Autodesk Inventor part; units mm, degrees
(part 4 of 4)
  line L152 (26.499495, -98.072286) -> (23.480041, -98.072286)
  line L153 (49.613875, -90.119995) -> (49.613875, -91.883884)
  line L154 (3.752764, -90.119995) -> (49.613875, -90.119995)
  line L155 (3.752764, -91.883884) -> (3.752764, -90.119995)
  line L156 (49.613875, -91.883884) -> (3.752764, -91.883884)
  line L157 (48.511932, -114.397733) -> (43.700857, -114.397733)
  spline S115 degree 3 poles (48.511932, -112.845889) (48.92121, -112.845889) (49.203363, -113.170245) (49.203363, -113.621725) (49.203363, -114.073205) (48.92121, -114.397733) (48.511932, -114.397733) knots 0 0 0 0 0.5 0.5 0.5 1 1 1 1
  line L158 (43.785606, -112.845889) -> (48.511932, -112.845889)
  spline S116 degree 3 poles (41.14718, -110.390914) (41.14718, -111.900555) (42.177091, -112.845889) (43.785606, -112.845889) knots 0 0 0 0 1 1 1 1
  spline S117 degree 3 poles (43.785606, -107.935939) (42.191216, -107.935939) (41.14718, -108.867148) (41.14718, -110.390914) knots 0 0 0 0 1 1 1 1
  line L159 (48.511932, -107.935939) -> (43.785606, -107.935939)
  spline S118 degree 3 poles (48.511932, -106.383924) (48.92121, -106.383924) (49.203363, -106.708452) (49.203363, -107.159931) (49.203363, -107.611411) (48.92121, -107.935939) (48.511932, -107.935939) knots 0 0 0 0 0.5 0.5 0.5 1 1 1 1
  line L160 (43.700857, -106.383924) -> (48.511932, -106.383924)
  spline S119 degree 3 poles (43.700857, -114.397733) (41.358881, -114.397733) (39.637539, -112.902217) (39.637539, -110.390914) (39.637539, -107.865487) (41.358881, -106.383924) (43.700857, -106.383924) knots 0 0 0 0 0.5 0.5 0.5 1 1 1 1
  spline S120 degree 3 poles (48.102827, -98.77767) (48.89296, -99.088073) (49.189238, -99.511303) (49.189238, -100.146234) knots 0 0 0 0 1 1 1 1
  line L161 (40.977853, -95.814887) -> (48.102827, -98.77767)
  spline S121 degree 3 poles (40.427671, -95.687763) (40.611123, -95.673811) (40.780449, -95.730138) (40.977853, -95.814887) knots 0 0 0 0 1 1 1 1
  spline S122 degree 3 poles (40.30072, -97.239779) (39.919692, -97.084577) (39.722288, -96.844799) (39.722288, -96.477896) (39.722288, -96.026416) (40.018566, -95.716013) (40.427671, -95.687763) knots 0 0 0 0 0.5 0.5 0.5 1 1 1 1
  line L162 (42.092514, -97.973412) -> (40.30072, -97.239779)
  line L163 (42.092514, -102.389508) -> (42.092514, -97.973412)
  line L164 (40.314844, -103.109016) -> (42.092514, -102.389508)
  spline S123 degree 3 poles (40.921526, -104.590407) (40.738074, -104.661031) (40.582873, -104.703406) (40.470046, -104.703406) (40.032691, -104.703406) (39.722288, -104.350628) (39.722288, -103.885024) (39.722288, -103.546371) (39.933817, -103.264217) (40.314844, -103.109016) knots 0 0 0 0 0.33333333 0.33333333 0.33333333 0.66666667 0.66666667 0.66666667 1 1 1 1
  line L165 (48.102827, -101.627625) -> (40.921526, -104.590407)
  spline S124 degree 3 poles (49.189238, -100.244936) (49.189238, -100.893992) (48.89296, -101.303097) (48.102827, -101.627625) knots 0 0 0 0 1 1 1 1
  line L166 (49.189238, -100.146234) -> (49.189238, -100.244936)
  line L167 (30.611044, -74.123016) -> (44.760051, -74.123016)
  line L168 (30.611044, -77.145915) -> (30.611044, -74.123016)
  line L169 (44.760051, -77.145915) -> (30.611044, -77.145915)
  line L170 (44.760051, -82.150088) -> (44.760051, -77.145915)
  line L171 (47.757456, -82.150088) -> (44.760051, -82.150088)
  line L172 (47.757456, -69.134173) -> (47.757456, -82.150088)
  line L173 (47.757456, -60.446504) -> (47.757456, -69.134173)
  spline S125 degree 3 poles (37.876061, -60.751395) (37.876061, -56.179064) (40.441624, -55.112118) (42.82942, -55.112118) (45.674552, -55.112118) (47.757456, -56.636228) (47.757456, -60.446504) knots 0 0 0 0 0.5 0.5 0.5 1 1 1 1
  line L174 (37.876061, -64.739609) -> (37.876061, -60.751395)
  spline S126 degree 3 poles (33.608449, -65.069822) (33.608449, -66.695562) (34.497628, -67.432124) (35.742341, -67.432124) (36.85993, -67.432124) (37.876061, -66.847836) (37.876061, -64.739609) knots 0 0 0 0 0.5 0.5 0.5 1 1 1 1
  line L175 (33.608449, -55.417009) -> (33.608449, -65.069822)
  line L176 (30.611044, -55.417009) -> (33.608449, -55.417009)
  line L177 (30.611044, -64.968192) -> (30.611044, -55.417009)
  spline S127 degree 3 poles (40.6957, -64.663301) (40.6957, -69.337262) (38.104643, -70.429701) (35.640711, -70.429701) (32.744764, -70.429701) (30.611044, -68.880097) (30.611044, -64.968192) knots 0 0 0 0 0.5 0.5 0.5 1 1 1 1
  line L178 (40.6957, -60.649764) -> (40.6957, -64.663301)
  spline S128 degree 3 poles (44.760051, -60.344873) (44.760051, -58.795442) (43.921859, -58.109523) (42.727962, -58.109523) (41.686337, -58.109523) (40.6957, -58.642996) (40.6957, -60.649764) knots 0 0 0 0 0.5 0.5 0.5 1 1 1 1
  line L179 (44.760051, -69.134173) -> (44.760051, -60.344873)
  line L180 (44.760051, -74.123016) -> (44.760051, -69.134173)
  line L181 (47.757456, -50.404739) -> (47.757456, -53.402317)
  line L182 (30.611044, -50.404739) -> (47.757456, -50.404739)
  line L183 (30.611044, -53.402317) -> (30.611044, -50.404739)
  line L184 (47.757456, -53.402317) -> (30.611044, -53.402317)
  line L185 (33.968117, -42.68115) -> (47.532836, -42.68115)
  spline S129 degree 3 poles (33.714042, -40.572752) (33.307692, -40.776012) (33.002802, -41.106225) (33.002802, -41.665019) (33.002802, -42.300123) (33.383829, -42.68115) (33.968117, -42.68115) knots 0 0 0 0 0.5 0.5 0.5 1 1 1 1
  line L186 (44.662383, -35.568578) -> (33.714042, -40.572752)
  spline S130 degree 3 poles (44.103588, -27.465197) (46.338938, -27.465197) (47.837727, -28.735231) (47.837727, -31.402596) (47.837727, -33.790392) (46.618508, -34.857166) (44.662383, -35.568578) knots 0 0 0 0 0.5 0.5 0.5 1 1 1 1
  line L187 (30.386424, -27.465197) -> (44.103588, -27.465197)
  line L188 (30.386424, -30.462602) -> (30.386424, -27.465197)
  line L189 (43.951143, -30.462602) -> (30.386424, -30.462602)
  spline S131 degree 3 poles (44.205219, -32.571001) (44.713198, -32.342419) (44.941952, -32.037528) (44.941952, -31.504055) (44.941952, -30.818308) (44.560925, -30.462602) (43.951143, -30.462602) knots 0 0 0 0 0.5 0.5 0.5 1 1 1 1
  line L190 (33.256877, -37.575346) -> (44.205219, -32.571001)
  spline S132 degree 3 poles (33.841166, -45.704049) (31.580322, -45.704049) (30.081533, -44.408521) (30.081533, -41.766649) (30.081533, -39.378854) (31.300924, -38.286586) (33.256877, -37.575346) knots 0 0 0 0 0.5 0.5 0.5 1 1 1 1
  line L191 (47.532836, -45.704049) -> (33.841166, -45.704049)
  line L192 (47.532836, -42.68115) -> (47.532836, -45.704049)
extrude "Extrusion1" add sketch "Sketch1 outline for Extrusion1" along normal blind 25.4
fillet "Fillet1" radius 12.7 4 edges at (-1.9102, 12.7, -1.9558) (-52.6889, 12.7, -25.6344) (-1.9102, 12.7, -192.4558) (-52.6889, 12.7, -216.1344)
body "Solid1"
